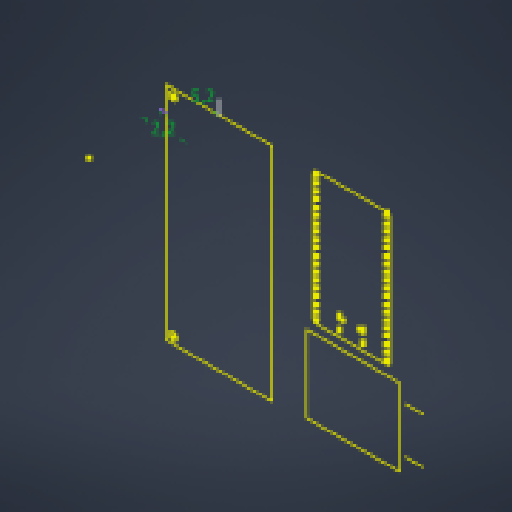
# Autodesk Inventor part: box_alert
Saved by Autodesk Inventor 2027.1 (Build 311270010, 270A)
## iProperties
Created: 2026-09-21
Part Number: box_alert
Material: Generic
Document SubType Name: Modeling
Designer: LENOVO
Density: 1 g/cm^3
Appearance: Default
Author: LENOVO
Autodesk Inventor part; units mm, degrees
ref_plane "YZ Plane" through (0, 0, 0) normal (1, 0, 0) x (0, 1, 0)
ref_plane "XZ Plane" through (0, 0, 0) normal (0, 1, 0) x (-1, 0, 0)
ref_plane "XY Plane" through (0, 0, 0) normal (0, 0, 1) x (1, 0, 0)
sketch "Sketch1" plane through (0, 0, 0) normal (0, 0, 1) x (1, 0, 0)
  line L0 (66.658361, -42.713186) -> (28.164225, -42.713186)
  line L1 (66.658361, 37.986814) -> (66.658361, -42.713186)
  line L2 (28.164225, 37.986814) -> (66.658361, 37.986814)
  line L3 (28.164225, -42.713186) -> (28.164225, 37.986814)
  ellipse E0 centre (30.663844, -40.213186) end of major axis (30.663844, -38.613186) minor radius 1.599756
  ellipse E1 centre (30.663844, 35.486814) end of major axis (30.663844, 37.086814) minor radius 1.599756
  line L4 (82.747581, 37.686486) -> (108.64504, 37.686486)
  arc A0 (82.747581, 37.686486) -> (81.760281, 36.699186) centre (82.747581, 36.699186) ccw
  line L5 (81.760281, -9.560911) -> (81.760281, 36.699186)
  arc A1 (81.760281, -9.560911) -> (82.747581, -10.548211) centre (82.747581, -9.560911) ccw
  line L6 (108.687637, -10.548211) -> (82.747581, -10.548211)
  arc A2 (108.687637, -10.548211) -> (109.674937, -9.560911) centre (108.687637, -9.560911) ccw
  line L7 (109.674937, 36.699186) -> (109.674937, -9.560911)
  arc A3 (109.674937, 36.699186) -> (108.729953, 37.685578) centre (108.687637, 36.699186) ccw
  arc A4 (108.64504, 37.686486) -> (108.729953, 37.685578) centre (108.687637, 37.699186) ccw
  circle A5 centre (82.992184, 36.449503) radius 0.524994
  circle A6 centre (82.992184, 33.909498) radius 0.524994
  circle A7 centre (82.992184, 28.829488) radius 0.524994
  circle A8 centre (82.992184, 31.369493) radius 0.524994
  circle A9 centre (82.992184, 11.049452) radius 0.524994
  circle A10 centre (82.992184, 8.509447) radius 0.524994
  circle A11 centre (82.992184, 5.969442) radius 0.524994
  circle A12 centre (82.992184, 3.429437) radius 0.524994
  circle A13 centre (82.992184, 23.749478) radius 0.524994
  circle A14 centre (82.992184, 21.209473) radius 0.524994
  circle A15 centre (82.992184, 18.669468) radius 0.524994
  circle A16 centre (82.992184, 13.589457) radius 0.524994
  circle A17 centre (82.992184, 16.129462) radius 0.524994
  circle A18 centre (82.992184, 0.889432) radius 0.524994
  circle A19 centre (82.992184, -1.650573) radius 0.524994
  circle A20 centre (82.992184, -4.190578) radius 0.524994
  circle A21 centre (82.992184, -6.730583) radius 0.524994
  circle A22 centre (82.992184, -9.270588) radius 0.524994
  circle A23 centre (82.992184, 26.289483) radius 0.524994
  line L8 (90.967088, -3.560771) -> (90.967088, -4.360797)
  arc A24 (91.767088, -3.560771) -> (90.967088, -3.560771) centre (91.367088, -3.560771) ccw
  line L9 (91.767088, -4.360797) -> (91.767088, -3.560771)
  arc A25 (90.967088, -4.360797) -> (91.767088, -4.360797) centre (91.367088, -4.360797) ccw
  line L10 (90.967088, -7.840616) -> (90.967088, -8.440616)
  arc A26 (91.767088, -7.840616) -> (90.967088, -7.840616) centre (91.367088, -7.840616) ccw
  line L11 (91.767088, -8.440616) -> (91.767088, -7.840616)
  arc A27 (90.967088, -8.440616) -> (91.767088, -8.440616) centre (91.367088, -8.440616) ccw
  circle A28 centre (92.792285, -4.460911) radius 0.375006
  circle A29 centre (98.592133, -4.460911) radius 0.375006
  line L12 (99.61733, -7.840616) -> (99.61733, -8.440616)
  arc A30 (100.41733, -7.840616) -> (99.61733, -7.840616) centre (100.01733, -7.840616) ccw
  line L13 (100.41733, -8.440616) -> (100.41733, -7.840616)
  arc A31 (99.61733, -8.440616) -> (100.41733, -8.440616) centre (100.01733, -8.440616) ccw
  line L14 (99.61733, -3.560797) -> (99.61733, -4.360771)
  arc A32 (100.41733, -3.560797) -> (99.61733, -3.560797) centre (100.01733, -3.560797) ccw
  line L15 (100.41733, -4.360771) -> (100.41733, -3.560797)
  arc A33 (99.61733, -4.360771) -> (100.41733, -4.360771) centre (100.01733, -4.360771) ccw
  circle A34 centre (108.399023, 11.042477) radius 0.524994
  circle A35 centre (108.399023, 8.502472) radius 0.524994
  circle A36 centre (108.399023, 16.122488) radius 0.524994
  circle A37 centre (108.399023, 18.662493) radius 0.524994
  circle A38 centre (108.399023, 21.202498) radius 0.524994
  circle A39 centre (108.399023, 23.742503) radius 0.524994
  circle A40 centre (108.399023, 13.582483) radius 0.524994
  circle A41 centre (108.399023, 26.282508) radius 0.524994
  circle A42 centre (108.399023, 5.962467) radius 0.524994
  circle A43 centre (108.399023, 3.422462) radius 0.524994
  circle A44 centre (108.399023, 0.882457) radius 0.524994
  circle A45 centre (108.399023, -4.197553) radius 0.524994
  circle A46 centre (108.399023, -1.657548) radius 0.524994
  circle A47 centre (108.399023, -6.737558) radius 0.524994
  circle A48 centre (108.399023, -9.277563) radius 0.524994
  circle A49 centre (108.399023, 36.442528) radius 0.524994
  circle A50 centre (108.399023, 33.902523) radius 0.524994
  circle A51 centre (108.399023, 28.822513) radius 0.524994
  circle A52 centre (108.399023, 31.362518) radius 0.524994
  line L16 (76.722886, -42.49753) -> (110.622886, -42.49753)
  line L17 (110.622886, -14.49753) -> (110.622886, -42.49753)
  line L18 (110.622886, -14.49753) -> (76.722886, -14.49753)
  line L19 (76.722886, -14.49753) -> (76.722886, -42.49753)
  line L20 (119.122886, -36.82253) -> (112.722886, -36.82253)
  line L21 (119.122886, -20.07253) -> (112.722886, -20.07253)
  line L22 (28.164225, 28.567894) -> (24.964225, 28.567894)
  line L23 (47.411293, 37.986814) -> (47.411293, 43.186814)
  line L24 (27.464225, 42.585579) -> (123.30779, 42.585579)
  line L25 (22.964225, 44.585579) -> (126.964225, 44.585579)
  line L26 (126.964225, 44.585579) -> (126.964225, -49.414421)
  line L27 (126.964225, -49.414421) -> (22.964225, -49.414421)
  line L28 (22.964225, -49.414421) -> (22.964225, 44.585579)
  line L29 (20.619985, -47.414421) -> (20.619985, -44.914421)
  line L30 (24.964225, -54.258028) -> (27.464225, -54.258028)
  arc A53 (27.464225, -47.414421) -> (24.964225, -44.914421) centre (25.552787, -46.825859) ccw
  line L31 (24.964225, -47.414421) -> (25.317778, -47.060868)
  circle A54 centre (25.317778, -47.060868) radius 1.35
  line L32 (24.964225, 48.233918) -> (27.464225, 48.233918)
  line L33 (20.619985, 42.585579) -> (20.619985, 40.085579)
  arc A55 (24.964225, 40.085579) -> (27.464225, 42.585579) centre (25.552787, 41.997016) ccw
  circle A56 centre (25.317778, 42.232025) radius 1.35
  line L34 (124.964225, 46.76255) -> (122.464225, 46.76255)
  line L35 (132.688253, 42.585579) -> (132.688253, 40.085579)
  arc A57 (122.464225, 42.585579) -> (124.964225, 40.085579) centre (124.375662, 41.997016) ccw
  circle A58 centre (124.610671, 42.232025) radius 1.35
  line L36 (133.638852, -47.414421) -> (133.638852, -44.914421)
  line L37 (124.964225, -54.782647) -> (122.464225, -54.782647)
  arc A59 (124.964225, -44.914421) -> (122.464225, -47.414421) centre (124.375662, -46.825859) ccw
  circle A60 centre (124.610671, -47.060868) radius 1.35
  line L38 (124.964225, 42.585579) -> (124.964225, 40.929144)
  line L39 (124.964225, 40.085579) -> (124.964225, -44.914421)
  line L40 (124.964225, -47.414421) -> (123.30779, -47.414421)
  line L41 (122.464225, -47.414421) -> (27.464225, -47.414421)
  line L42 (26.620659, -47.414421) -> (24.964225, -47.414421)
  line L43 (24.964225, -47.414421) -> (24.964225, -45.757987)
  line L44 (24.964225, -44.914421) -> (24.964225, 40.085579)
  point P0 (0, 0)
  dimension "d0" = 3.2
  dimension "d1" = 5.2
  dimension "d4" = 90
  dimension "d9" = 2.5
  dimension "d13" = 2.5
  dimension "d14" = 2
  dimension "d16" = 0.5
  dimension "d17" = 2.7
  dimension "d18" = 2.5
  dimension "d19" = 2.5
  dimension "d20" = 2
  dimension "d22" = 2.7
  dimension "d23" = 2.5
  dimension "d24" = 2.5
  dimension "d25" = 2
  dimension "d27" = 2.7
  dimension "d28" = 2.5
  dimension "d29" = 2.5
  dimension "d31" = 2
  constraints: 46 end point, 12 point on circle, 9 parallel, 7 centre point, 7 horizontal, 5 vertical, 3 perpendicular, 2 point on line, 1 coincident, 1 midpoint, 5 other
  measures "d0" distance of L22.start L22.end
  measures "d1" distance of L23.start L23.end
  measures "d4" distance of L38.start L40.start
  measures "d9" distance of L29.start L29.end
  measures "d13" distance of L30.start L30.end
  measures "d14" radius of A53
  measures "d16" distance of L31.start L31.end
  measures "d17" diameter of A54
  measures "d18" distance of L32.start L32.end
  measures "d19" distance of L33.start L33.end
  measures "d20" radius of A55
  measures "d22" diameter of A56
  measures "d23" distance of L34.start L34.end
  measures "d24" distance of L35.start L35.end
  measures "d25" radius of A57
  measures "d27" diameter of A58
  measures "d28" distance of L36.start L36.end
  measures "d29" distance of L37.start L37.end
  measures "d31" radius of A59
extrude "Extrusion1" add sketch "Sketch1" along normal blind 70 contours L25 L26 L27 L28
sketch "Sketch2" plane through (126.964225, -49.414421, 0) normal (1, 0, 0) x (0, 0, -1)
  line L0 (0, 0) -> (0, 94) projected
  line L1 (0, 94) -> (-70, 94) projected
  line L2 (-70, 0) -> (-70, 94) projected
  line L3 (0, 0) -> (-70, 0) projected
  line L4 (0, 94) -> (-2, 94)
  line L5 (-2, 94) -> (-2, 0)
  line L6 (-2, 0) -> (0, 0)
  line L7 (0, 0) -> (0, 94)
  point P0 (0, 49.414421)
  dimension "d35" = 2
  constraints: 8 end point, 2 parallel, 1 horizontal, 1 perpendicular, 1 point on line
  measures "d35" distance of L6.end L5.end
sketch "Sketch3" plane through (0, 0, 0) normal (0, 0, -1) x (-1, 0, 0)
  circle A0 centre (-124.610671, 42.232025) radius 1.35
  circle A1 centre (-25.317778, 42.232025) radius 1.35
  circle A2 centre (-25.317778, -47.060868) radius 1.35
  circle A3 centre (-124.610671, -47.060868) radius 1.35
  point P0 (0, 0)
extrude "Extrusion2" add sketch "Sketch3" against normal blind 63
extrude "Extrusion3" add sketch "Sketch2" against normal blind 104 contours L3 L5 L1 L0
sketch "Sketch4" plane through (27.464225, 42.585579, 2) normal (0, 0, 1) x (1, 0, 0)
  line L0 (39.194136, -85.298765) -> (0.7, -85.298765)
  line L1 (39.194136, -4.598765) -> (39.194136, -85.298765)
  line L2 (0.7, -4.598765) -> (39.194136, -4.598765)
  line L3 (0.7, -85.298765) -> (0.7, -4.598765)
  ellipse E0 centre (3.199619, -82.798765) end of major axis (3.199619, -81.198765) minor radius 1.599756
  ellipse E1 centre (3.199619, -7.098765) end of major axis (3.199619, -5.498765) minor radius 1.599756
  line L4 (0.7, -4.116878) -> (6.7, -4.116878)
  line L5 (0.196118, -4.66095) -> (0.196118, -10.66095)
  arc A0 (0.7, -10.66095) -> (6.685165, -4.598765) centre (1.829171, -5.790121) ccw
  line L6 (0.7, -85.91832) -> (6.7, -85.91832)
  line L7 (0.32353, -85.36095) -> (0.32353, -79.36095)
  arc A1 (6.713999, -85.298765) -> (0.7, -79.36095) centre (1.829171, -84.231779) ccw
  line L8 (55.283357, -4.899093) -> (81.180815, -4.899093)
  arc A2 (55.283357, -4.899093) -> (54.296057, -5.886393) centre (55.283357, -5.886393) ccw
  line L9 (54.296057, -52.14649) -> (54.296057, -5.886393)
  arc A3 (54.296057, -52.14649) -> (55.283357, -53.133789) centre (55.283357, -52.14649) ccw
  line L10 (81.223412, -53.133789) -> (55.283357, -53.133789)
  arc A4 (81.223412, -53.133789) -> (82.210712, -52.14649) centre (81.223413, -52.14649) ccw
  line L11 (82.210712, -5.886393) -> (82.210712, -52.14649)
  arc A5 (82.210712, -5.886393) -> (81.265729, -4.9) centre (81.223413, -5.886393) ccw
  arc A6 (81.180815, -4.899093) -> (81.265729, -4.9) centre (81.223412, -4.886393) ccw
  circle A7 centre (55.527959, -6.136075) radius 0.524994
  circle A8 centre (55.527959, -8.676081) radius 0.524994
  circle A9 centre (55.527959, -13.756091) radius 0.524994
  circle A10 centre (55.527959, -11.216086) radius 0.524994
  circle A11 centre (55.527959, -31.536126) radius 0.524994
  circle A12 centre (55.527959, -34.076131) radius 0.524994
  circle A13 centre (55.527959, -36.616136) radius 0.524994
  circle A14 centre (55.527959, -39.156142) radius 0.524994
  circle A15 centre (55.527959, -18.836101) radius 0.524994
  circle A16 centre (55.527959, -21.376106) radius 0.524994
  circle A17 centre (55.527959, -23.916111) radius 0.524994
  circle A18 centre (55.527959, -28.996121) radius 0.524994
  circle A19 centre (55.527959, -26.456116) radius 0.524994
  circle A20 centre (55.527959, -41.696147) radius 0.524994
  circle A21 centre (55.527959, -44.236152) radius 0.524994
  circle A22 centre (55.527959, -46.776157) radius 0.524994
  circle A23 centre (55.527959, -49.316162) radius 0.524994
  circle A24 centre (55.527959, -51.856167) radius 0.524994
  circle A25 centre (55.527959, -16.296096) radius 0.524994
  line L12 (63.502864, -46.14635) -> (63.502864, -46.946375)
  arc A26 (64.302864, -46.14635) -> (63.502864, -46.14635) centre (63.902864, -46.14635) ccw
  line L13 (64.302864, -46.946375) -> (64.302864, -46.14635)
  arc A27 (63.502864, -46.946375) -> (64.302864, -46.946375) centre (63.902864, -46.946375) ccw
  line L14 (63.502864, -50.426195) -> (63.502864, -51.026195)
  arc A28 (64.302864, -50.426195) -> (63.502864, -50.426195) centre (63.902864, -50.426195) ccw
  line L15 (64.302864, -51.026195) -> (64.302864, -50.426195)
  arc A29 (63.502864, -51.026195) -> (64.302864, -51.026195) centre (63.902864, -51.026195) ccw
  circle A30 centre (65.328061, -47.04649) radius 0.375006
  circle A31 centre (71.127908, -47.04649) radius 0.375006
  line L16 (72.153105, -50.426195) -> (72.153105, -51.026195)
  arc A32 (72.953105, -50.426195) -> (72.153105, -50.426195) centre (72.553105, -50.426195) ccw
  line L17 (72.953105, -51.026195) -> (72.953105, -50.426195)
  arc A33 (72.153105, -51.026195) -> (72.953105, -51.026195) centre (72.553105, -51.026195) ccw
  line L18 (72.153105, -46.146375) -> (72.153105, -46.94635)
  arc A34 (72.953105, -46.146375) -> (72.153105, -46.146375) centre (72.553105, -46.146375) ccw
  line L19 (72.953105, -46.94635) -> (72.953105, -46.146375)
  arc A35 (72.153105, -46.94635) -> (72.953105, -46.94635) centre (72.553105, -46.94635) ccw
  circle A36 centre (80.934799, -31.543101) radius 0.524994
  circle A37 centre (80.934799, -34.083106) radius 0.524994
  circle A38 centre (80.934799, -26.463091) radius 0.524994
  circle A39 centre (80.934799, -23.923086) radius 0.524994
  circle A40 centre (80.934799, -21.383081) radius 0.524994
  circle A41 centre (80.934799, -18.843076) radius 0.524994
  circle A42 centre (80.934799, -29.003096) radius 0.524994
  circle A43 centre (80.934799, -16.303071) radius 0.524994
  circle A44 centre (80.934799, -36.623111) radius 0.524994
  circle A45 centre (80.934799, -39.163116) radius 0.524994
  circle A46 centre (80.934799, -41.703121) radius 0.524994
  circle A47 centre (80.934799, -46.783132) radius 0.524994
  circle A48 centre (80.934799, -44.243127) radius 0.524994
  circle A49 centre (80.934799, -49.323137) radius 0.524994
  circle A50 centre (80.934799, -51.863142) radius 0.524994
  circle A51 centre (80.934799, -6.14305) radius 0.524994
  circle A52 centre (80.934799, -8.683055) radius 0.524994
  circle A53 centre (80.934799, -13.763066) radius 0.524994
  circle A54 centre (80.934799, -11.22306) radius 0.524994
  point P0 (-27.464225, -42.585579)
  dimension "d40" = 6
  dimension "d41" = 6
  dimension "d42" = 5
  dimension "d43" = 6
  dimension "d44" = 6
  dimension "d45" = 5
  constraints: 8 end point, 4 point on circle, 4 point on line, 2 centre point, 2 horizontal, 2 vertical, 2 other
  measures "d40" distance of L4.start L4.end
  measures "d41" distance of L5.start L5.end
  measures "d42" radius of A0
  measures "d43" distance of L6.start L6.end
  measures "d44" distance of L7.start L7.end
  measures "d45" radius of A1
extrude "Extrusion4" add sketch "Sketch4" along normal blind 27 contours L0 L3 A1 | A0 L3 L2
sketch "Sketch5" plane through (27.464225, 42.585579, 2) normal (0, 0, 1) x (1, 0, 0)
  line L0 (55.283357, -4.899093) -> (81.180815, -4.899093)
  arc A0 (55.283357, -4.899093) -> (54.296057, -5.886393) centre (55.283357, -5.886393) ccw
  line L1 (54.296057, -52.14649) -> (54.296057, -5.886393)
  arc A1 (54.296057, -52.14649) -> (55.283357, -53.133789) centre (55.283357, -52.14649) ccw
  line L2 (81.223412, -53.133789) -> (55.283357, -53.133789)
  arc A2 (81.223412, -53.133789) -> (82.210712, -52.14649) centre (81.223413, -52.14649) ccw
  line L3 (82.210712, -5.886393) -> (82.210712, -52.14649)
  arc A3 (82.210712, -5.886393) -> (81.265729, -4.9) centre (81.223413, -5.886393) ccw
  arc A4 (81.180815, -4.899093) -> (81.265729, -4.9) centre (81.223412, -4.886393) ccw
  circle A5 centre (55.527959, -6.136075) radius 0.524994
  circle A6 centre (55.527959, -8.676081) radius 0.524994
  circle A7 centre (55.527959, -13.756091) radius 0.524994
  circle A8 centre (55.527959, -11.216086) radius 0.524994
  circle A9 centre (55.527959, -31.536126) radius 0.524994
  circle A10 centre (55.527959, -34.076131) radius 0.524994
  circle A11 centre (55.527959, -36.616136) radius 0.524994
  circle A12 centre (55.527959, -39.156142) radius 0.524994
  circle A13 centre (55.527959, -18.836101) radius 0.524994
  circle A14 centre (55.527959, -21.376106) radius 0.524994
  circle A15 centre (55.527959, -23.916111) radius 0.524994
  circle A16 centre (55.527959, -28.996121) radius 0.524994
  circle A17 centre (55.527959, -26.456116) radius 0.524994
  circle A18 centre (55.527959, -41.696147) radius 0.524994
  circle A19 centre (55.527959, -44.236152) radius 0.524994
  circle A20 centre (55.527959, -46.776157) radius 0.524994
  circle A21 centre (55.527959, -49.316162) radius 0.524994
  circle A22 centre (55.527959, -51.856167) radius 0.524994
  circle A23 centre (55.527959, -16.296096) radius 0.524994
  line L4 (63.502864, -46.14635) -> (63.502864, -46.946375)
  arc A24 (64.302864, -46.14635) -> (63.502864, -46.14635) centre (63.902864, -46.14635) ccw
  line L5 (64.302864, -46.946375) -> (64.302864, -46.14635)
  arc A25 (63.502864, -46.946375) -> (64.302864, -46.946375) centre (63.902864, -46.946375) ccw
  line L6 (63.502864, -50.426195) -> (63.502864, -51.026195)
  arc A26 (64.302864, -50.426195) -> (63.502864, -50.426195) centre (63.902864, -50.426195) ccw
  line L7 (64.302864, -51.026195) -> (64.302864, -50.426195)
  arc A27 (63.502864, -51.026195) -> (64.302864, -51.026195) centre (63.902864, -51.026195) ccw
  circle A28 centre (65.328061, -47.04649) radius 0.375006
  circle A29 centre (71.127908, -47.04649) radius 0.375006
  line L8 (72.153105, -50.426195) -> (72.153105, -51.026195)
  arc A30 (72.953105, -50.426195) -> (72.153105, -50.426195) centre (72.553105, -50.426195) ccw
  line L9 (72.953105, -51.026195) -> (72.953105, -50.426195)
  arc A31 (72.153105, -51.026195) -> (72.953105, -51.026195) centre (72.553105, -51.026195) ccw
  line L10 (72.153105, -46.146375) -> (72.153105, -46.94635)
  arc A32 (72.953105, -46.146375) -> (72.153105, -46.146375) centre (72.553105, -46.146375) ccw
  line L11 (72.953105, -46.94635) -> (72.953105, -46.146375)
  arc A33 (72.153105, -46.94635) -> (72.953105, -46.94635) centre (72.553105, -46.94635) ccw
  circle A34 centre (80.934799, -31.543101) radius 0.524994
  circle A35 centre (80.934799, -34.083106) radius 0.524994
  circle A36 centre (80.934799, -26.463091) radius 0.524994
  circle A37 centre (80.934799, -23.923086) radius 0.524994
  circle A38 centre (80.934799, -21.383081) radius 0.524994
  circle A39 centre (80.934799, -18.843076) radius 0.524994
  circle A40 centre (80.934799, -29.003096) radius 0.524994
  circle A41 centre (80.934799, -16.303071) radius 0.524994
  circle A42 centre (80.934799, -36.623111) radius 0.524994
  circle A43 centre (80.934799, -39.163116) radius 0.524994
  circle A44 centre (80.934799, -41.703121) radius 0.524994
  circle A45 centre (80.934799, -46.783132) radius 0.524994
  circle A46 centre (80.934799, -44.243127) radius 0.524994
  circle A47 centre (80.934799, -49.323137) radius 0.524994
  circle A48 centre (80.934799, -51.863142) radius 0.524994
  circle A49 centre (80.934799, -6.14305) radius 0.524994
  circle A50 centre (80.934799, -8.683055) radius 0.524994
  circle A51 centre (80.934799, -13.763066) radius 0.524994
  circle A52 centre (80.934799, -11.22306) radius 0.524994
  line L12 (63.902864, -16.303071) -> (72.902864, -16.303071)
  line L13 (72.902864, -16.303071) -> (72.902864, -42.303071)
  line L14 (72.902864, -42.303071) -> (63.902864, -42.303071)
  line L15 (63.902864, -42.303071) -> (63.902864, -16.303071)
  point P0 (-27.464225, -42.585579)
  dimension "d50" = 9
  dimension "d51" = 26
  constraints: 8 end point, 2 parallel, 1 horizontal, 1 perpendicular
  measures "d50" distance of L13.end L14.end
  measures "d51" distance of L12.end L13.end
extrude "Extrusion5" add sketch "Sketch5" along normal blind 26 contours L12 L13 L14 L15
sketch "Sketch6" plane through (27.464225, 42.585579, 2) normal (0, 0, 1) x (1, 0, 0)
  line L0 (49.258662, -85.083109) -> (83.158662, -85.083109)
  line L1 (83.158662, -57.083109) -> (83.158662, -85.083109)
  line L2 (83.158662, -57.083109) -> (49.258662, -57.083109)
  line L3 (49.258662, -57.083109) -> (49.258662, -85.083109)
  line L4 (91.658662, -62.658109) -> (85.258662, -62.658109)
  line L5 (91.658662, -79.408109) -> (85.258662, -79.408109)
  line L6 (63.902864, -42.303071) -> (63.902864, -16.303071)
  line L7 (63.902864, -16.303071) -> (72.902864, -16.303071)
  line L8 (72.902864, -16.303071) -> (72.902864, -42.303071)
  line L9 (72.902864, -42.303071) -> (63.902864, -42.303071)
  arc A0 (6.713999, -85.298765) -> (0.7, -79.36095) centre (1.829171, -84.231779) ccw
  line L10 (6.713999, -85.298765) -> (0.7, -85.298765)
  line L11 (0.7, -85.298765) -> (0.7, -79.36095)
  arc A1 (0.7, -10.66095) -> (6.685165, -4.598765) centre (1.829171, -5.790121) ccw
  line L12 (0.7, -10.66095) -> (0.7, -4.598765)
  line L13 (0.7, -4.598765) -> (6.685165, -4.598765)
  line L14 (0, 0) -> (95, 0)
  arc A2 (-2.5, -2.5) -> (0, 0) centre (-1.911438, -0.588562) ccw
  line L15 (-2.5, -87.5) -> (-2.5, -2.5)
  arc A3 (0, -90) -> (-2.5, -87.5) centre (-1.911438, -89.411438) ccw
  line L16 (95, -90) -> (0, -90)
  arc A4 (97.5, -87.5) -> (95, -90) centre (96.911438, -89.411438) ccw
  line L17 (97.5, -2.5) -> (97.5, -87.5)
  arc A5 (95, 0) -> (97.5, -2.5) centre (96.911438, -0.588562) ccw
  line L18 (46.505431, -56.083109) -> (46.505431, -76.580215)
  line L19 (46.505431, -56.083109) -> (97.5, -56.083109)
  line L20 (45.005431, -55.083109) -> (45.005431, -76.580215)
  line L21 (45.005431, -55.083109) -> (97.5, -55.083109)
  line L22 (45.005431, -76.580215) -> (46.505431, -76.580215)
  point P0 (-27.464225, -42.585579)
  constraints: 10 end point, 5 perpendicular, 2 point on line
extrude "Extrusion6" add sketch "Sketch6" along normal blind 18 contours L17 L19 L18 L22 L20 L21
sketch "Sketch7" plane through (0, 0, 70) normal (0, 0, 1) x (1, 0, 0)
  line L0 (22.964225, -49.414421) -> (126.964225, -49.414421)
  line L1 (126.964225, -49.414421) -> (126.964225, 44.585579)
  line L2 (126.964225, 44.585579) -> (22.964225, 44.585579)
  line L3 (22.964225, 44.585579) -> (22.964225, -49.414421)
  circle A0 centre (124.610671, 42.232025) radius 1.35
  circle A1 centre (124.610671, -47.060868) radius 1.35
  circle A2 centre (25.317778, -47.060868) radius 1.35
  circle A3 centre (25.317778, 42.232025) radius 1.35
  arc A4 (122.464225, 42.585579) -> (124.964225, 40.085579) centre (124.375662, 41.997016) ccw
  line L4 (124.964225, 40.085579) -> (124.964225, -44.914421)
  arc A5 (124.964225, -44.914421) -> (122.464225, -47.414421) centre (124.375662, -46.825859) ccw
  line L5 (122.464225, -47.414421) -> (27.464225, -47.414421)
  arc A6 (27.464225, -47.414421) -> (24.964225, -44.914421) centre (25.552787, -46.825859) ccw
  line L6 (24.964225, -44.914421) -> (24.964225, 40.085579)
  arc A7 (24.964225, 40.085579) -> (27.464225, 42.585579) centre (25.552787, 41.997016) ccw
  line L7 (27.464225, 42.585579) -> (122.464225, 42.585579)
  line L8 (24.964225, 40.085579) -> (21.028203, 40.085579)
  line L9 (27.464225, 42.585579) -> (27.464225, 45.564858)
  line L10 (122.464225, 42.585579) -> (122.464225, 47.935687)
  line L11 (124.964225, 40.085579) -> (129.99491, 40.085579)
  line L12 (124.964225, -44.914421) -> (128.814326, -44.914421)
  line L13 (122.464225, -47.414421) -> (122.464225, -50.977125)
  line L14 (27.464225, -47.414421) -> (27.464225, -51.779087)
  arc A8 (27.464225, -47.414421) -> (24.964225, -44.914421) centre (25.552787, -46.825859) ccw
  line L15 (24.964225, -44.914421) -> (19.333314, -44.914421)
  line L16 (124.964225, -26.750429) -> (125.964225, -26.750429)
  line L17 (74.964225, 42.585579) -> (74.964225, 43.585579)
  line L18 (24.964225, -2.414421) -> (23.964225, -2.414421)
  line L19 (27.464225, -48.414421) -> (122.464225, -48.414421)
  line L20 (125.964225, -44.914421) -> (125.964225, 40.085579)
  line L21 (122.464225, 43.585579) -> (27.464225, 43.585579)
  line L22 (23.964225, 40.085579) -> (23.964225, -44.914421)
  point P0 (0, 0)
  point P1 (22.964225, 40.085579)
  point P2 (22.964225, -44.914421)
  point P3 (122.464225, 44.585579)
  point P4 (27.464225, 44.585579)
  point P5 (126.964225, -44.914421)
  point P6 (126.964225, 40.085579)
  point P7 (27.464225, -49.414421)
  point P8 (122.464225, -49.414421)
  dimension "d69" = 1
  dimension "d70" = 1
  dimension "d71" = 1
  constraints: 30 end point, 9 point on line, 6 perpendicular, 4 horizontal, 4 vertical, 2 midpoint, 1 parallel
  measures "d69" distance of L16.start L16.end
  measures "d70" distance of L17.start L17.end
  measures "d71" distance of L18.start L18.end
extrude "Extrusion7" cut sketch "Sketch7" against normal blind 4 contours L14 L19 L13 L0 | L3 L8 L22 L15 | L12 L20 L11 L1 | L2 L10 L21 L9
fillet "Fillet1" radius 1.5 4 edges at (126.9642, -49.4144, 35) (126.9642, 44.5856, 35) (22.9642, 44.5856, 35) (22.9642, -49.4144, 35)
sketch "Sketch8" plane through (126.964225, -44.914421, 66) normal (1, 0, 0) x (0, 0, -1)
  line L0 (-4, 88) -> (66, 88)
  line L1 (-4, 85) -> (-4, 88)
  line L2 (-4, 85) -> (0, 85)
  line L3 (0, 85) -> (0, 0)
  line L4 (0, 0) -> (-4, 0)
  line L5 (-4, -3) -> (-4, 0)
  line L6 (66, -3) -> (-4, -3)
  line L7 (66, -3) -> (66, 88)
  circle A0 centre (15.485479, 59.924767) radius 3.1
  point P0 (66, 44.914421)
  dimension "d75" = 6.2
  constraints: 1 centre point
  measures "d75" diameter of A0
extrude "Extrusion8" cut sketch "Sketch8" against normal blind 4 contours A0
thread "Thread1" size "M6x0.75" class "6H" standard "ANSI Metric M Profile" full length
sketch "Sketch9" plane through (27.464225, -49.414421, 66) normal (0, -1, 0) x (1, 0, 0)
  circle A0 centre (17.880603, -17.019131) radius 3.9
  point P0 (-27.464225, -66)
  dimension "d80" = 7.8
  constraints: 1 centre point
  measures "d80" diameter of A0
extrude "Extrusion9" cut sketch "Sketch9" against normal blind 4
sketch "Sketch10" plane through (22.964225, -44.914421, 66) normal (-1, 0, 0) x (0, 0, 1)
  ellipse E0 centre (-32.735386, 60.034958) end of major axis (-34.055386, 60.034958) minor radius 1.319943 (-31.415386, 60.034958) -> (-34.055386, 60.034958) ccw
  ellipse E1 centre (-32.735386, 54.255208) end of major axis (-31.415386, 54.255208) minor radius 1.319943 (-34.055386, 54.255208) -> (-31.415386, 54.255208) ccw
  line L0 (-31.415386, 60.034958) -> (-31.415386, 54.255208)
  line L1 (-31.415386, 60.034958) -> (-29.415386, 60.034958)
  line L2 (-34.055386, 60.034958) -> (-36.055386, 60.034958)
  line L3 (-34.055386, 54.255208) -> (-36.055386, 54.255208)
  line L4 (-36.055385, 61.534958) -> (-36.055385, 52.755208)
  line L5 (-29.415385, 52.755208) -> (-29.415385, 61.534958)
  arc A0 (-29.415386, 60.034958) -> (-36.055386, 60.034958) centre (-32.735386, 60.071251) ccw
  arc A1 (-36.055386, 54.255208) -> (-29.415385, 54.257435) centre (-32.735386, 54.257435) ccw
  line L6 (-29.415385, 61.534958) -> (-29.755238, 61.534958)
  line L7 (-35.715534, 61.534958) -> (-36.055385, 61.534958)
  line L8 (-36.055385, 52.755208) -> (-35.696082, 52.755208)
  line L9 (-29.77469, 52.755208) -> (-29.415385, 52.755208)
  point P0 (-66, 44.914421)
  point P1 (-36.055385, 54.254286)
  point P2 (-29.415385, 60.107477)
  point P3 (-36.055385, 60.107613)
  dimension "d83" = 2
  dimension "d84" = 2
  dimension "d86" = 2
  dimension "d90" = 3.3202
  constraints: 18 end point, 8 point on circle, 5 horizontal, 5 parallel, 2 centre point, 2 perpendicular, 1 point on line, 1 tangent, 2 other
  measures "d83" distance of L0.start L1.end
  measures "d84" distance of L2.start L2.end
  measures "d86" distance of L3.start L3.end
  measures "d90" radius of A0
sketch "Sketch10 outline for Extrusion10" plane through (22.964225, -44.914421, 66) normal (-1, 0, 0) x (0, 0, 1)
  line L0 (-36.055385, 60.107613) -> (-36.055385, 54.254286)
  arc A0 (-29.415385, 60.107477) -> (-36.055385, 60.107613) centre (-32.735386, 60.071251) ccw
  line L1 (-29.415385, 54.257435) -> (-29.415385, 60.107477)
  arc A1 (-36.055385, 54.254286) -> (-29.415385, 54.257435) centre (-32.735386, 54.257435) ccw
extrude "Extrusion10" cut sketch "Sketch10 outline for Extrusion10" against normal blind 4
body "Solid1"
